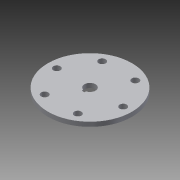
# Autodesk Inventor part: Pneumatic Hub
Saved by Autodesk Inventor 2014 SP1 (Build 180222100, 222)
## iProperties
Created: 2013-01-19
Part Number: Pneumatic Hub
Material: Aluminum 6061
Document SubType Name: Modeling
Designer: actoennies
Density: 2.71 g/cm^3
Mass: 23.0954 g
Surface Area: 63.61 cm^2
Volume: 8.5223 cm^3
Appearance: Aluminum - Flat
Author: actoennies
Autodesk Inventor part; units mm, degrees
ref_plane "YZ Plane" through (0, 0, 0) normal (1, 0, 0) x (0, 1, 0)
ref_plane "XZ Plane" through (0, 0, 0) normal (0, 1, 0) x (-1, 0, 0)
ref_plane "XY Plane" through (0, 0, 0) normal (0, 0, 1) x (1, 0, 0)
sketch "Sketch1" plane through (0, 0, 0) normal (0, 1, 0) x (-1, 0, 0)
  circle A0 centre (-23.8125, 0) radius 2.54
  circle A1 centre (-11.9063, 20.6222) radius 2.54
  circle A2 centre (11.9062, 20.6222) radius 2.54
  circle A3 centre (23.8125, 0) radius 2.54
  circle A4 centre (-11.9063, -20.6222) radius 2.54
  circle A5 centre (11.9062, -20.6222) radius 2.54
  circle A6 centre (0, 0) radius 30.1625
  arc A7 (-1, 3.873) -> (1, 3.873) centre (0, 0) ccw
  line L0 (1, 3.873) -> (1, 5)
  line L1 (1, 5) -> (-1, 5)
  line L2 (-1, 5) -> (-1, 3.873)
  dimension "d0" = 5.08
  dimension "d6" = 5.08
  dimension "d8" = 5.08
  dimension "d10" = 5.08
  dimension "d11" = 60.325
  dimension "d15" = 8
  dimension "d19" = 1
  dimension "d20" = 1
  dimension "d22" = 0
  dimension "d23" = 1
  constraints: 8 centre point, 6 end point, 2 coincident, 2 point on circle, 1 parallel, 1 perpendicular, 1 vertical, 2 other
  measures "d0" diameter of A0
  measures "d6" diameter of A1
  measures "d8" diameter of A3
  measures "d10" diameter of A4
  measures "d11" diameter of A6
  measures "d15" diameter of A7
  measures "d19" distance from line of point (0, 0) L0
  measures "d20" distance from line of point (0, 0) L2
  measures "d22" distance of point (0, 0) point (0, 0)
  measures "d23" distance edge to line of A7 L1
extrude "Extrusion2" add sketch "Sketch1" along normal blind 3.175
body "Solid2"
